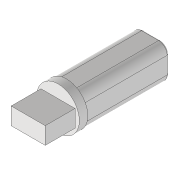
# Autodesk Inventor part: Hubvorrichtung
Saved by Autodesk Inventor 2020 (Build 240168000, 168)
## iProperties
Created: 2020-03-18
Part Number: Hubvorrichtung
Material: Generisch
Document SubType Name: Modeling
Designer: franz
Density: 1 g/cm^3
Appearance: Vorgabe
Author: franz
Autodesk Inventor part; units mm, degrees
ref_plane "YZ Plane" through (0, 0, 0) normal (1, 0, 0) x (0, 1, 0)
ref_plane "XZ Plane" through (0, 0, 0) normal (0, 1, 0) x (-1, 0, 0)
ref_plane "XY Plane" through (0, 0, 0) normal (0, 0, 1) x (1, 0, 0)
sketch "Skizze2" plane through (0, 0, 0) normal (0, 0, 1) x (1, 0, 0)
  line L0 (-20, -10) -> (20, -10)
  line L1 (20, -10) -> (20, 10)
  line L2 (20, 10) -> (-20, 10)
  line L3 (-20, 10) -> (-20, -10)
  line L4 (-20, -10) -> (20, 10) construction
  line L5 (20, -10) -> (-20, 10) construction
  point P0 (0, 0)
  dimension "d0" = 40
  dimension "d1" = 20
  constraints: 12 end point, 2 midpoint, 2 parallel, 1 horizontal, 1 perpendicular
  measures "d0" distance of L2.end L1.end
  measures "d1" distance of L1.end L0.end
extrude "Extrusion1" add sketch "Skizze2" along normal blind 35
sketch "Skizze3" plane through (0, 0, 0) normal (0, 0, -1) x (-1, 0, 0)
  circle A0 centre (0, 0) radius 25
  dimension "d4" = 50
  constraints: 1 centre point, 1 coincident
  measures "d4" diameter of A0
extrude "Extrusion2" add sketch "Skizze3" along normal blind 10
sketch "Skizze4" plane through (0, 0, -10) normal (0, 0, -1) x (-1, 0, 0)
  line L0 (10, -20) -> (-10, -20)
  line L1 (-20, -10) -> (-20, 10)
  line L2 (-10, 20) -> (10, 20)
  line L3 (20, 10) -> (20, -10)
  line L4 (20, -20) -> (-20, 20) construction
  line L5 (-20, -20) -> (20, 20) construction
  arc A0 (-20, -10) -> (-10, -20) centre (-10, -10) ccw
  arc A1 (-10, 20) -> (-20, 10) centre (-10, 10) ccw
  arc A2 (20, 10) -> (10, 20) centre (10, 10) ccw
  arc A3 (10, -20) -> (20, -10) centre (10, -10) ccw
  point P0 (0, 0)
  dimension "d7" = 40
  dimension "d8" = 40
  dimension "d9" = 10
  constraints: 12 end point, 8 point on circle, 8 point on line, 8 tangent, 4 centre point, 3 equal radius, 2 midpoint, 2 parallel, 1 horizontal, 1 perpendicular
  measures "d7" distance of L4.end L5.end
  measures "d8" distance of L5.start L4.end
  measures "d9" radius of A0
extrude "Extrusion3" add sketch "Skizze4" along normal blind 100
sketch "Skizze5" plane through (0, 0, -110) normal (0, 0, -1) x (-1, 0, 0)
  circle A0 centre (0, 0) radius 10
  dimension "d12" = 20
  constraints: 1 centre point, 1 coincident
  measures "d12" diameter of A0
extrude "Extrusion4" cut sketch "Skizze5" against normal up to surface (100 mm away)
fillet "Rundung1" radius 2 9 edges at (17.0711, -17.0711, -110) (0, -20, -110) (-17.0711, -17.0711, -110) (-20, 0, -110) (-17.0711, 17.0711, -110) (0, 20, -110) (17.0711, 17.0711, -110) (20, 0, -110) (10, 0, -110)
